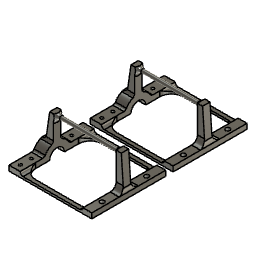
Amemometer_case v2 (Autodesk Fusion 360 design; units mm, degrees)
Autodesk Fusion 360 part; units mm, degrees
sketch "Sketch1" plane through (0, 0, 0) normal (0, 0, 1) x (1, 0, 0)
  arc A0 (0, 10) -> (0, -10) centre (0, 0) ccw
  line L0 (0, -10) -> (0, -50)
  line L1 (0, -50) -> (-7, -50)
  line L2 (-7, -50) -> (-7, -17)
  line L3 (0, 10) -> (0, 50)
  line L4 (0, 50) -> (-7, 50)
  line L5 (-7, 50) -> (-7, 17)
  line L6 (-52, -5) -> (-17.6918, -5)
  line L7 (-52, -5) -> (-52, 5)
  line L8 (-52, 5) -> (-17.6918, 5)
  arc A1 (-17.6918, -5) -> (-7, -17) centre (0, 0) ccw
  arc A2 (-7, 17) -> (-17.6918, 5) centre (0, 0) ccw
  dimension "d2" = 40
  dimension "d3" = 40
  dimension "d5" = 7
  dimension "d8" = 7
  dimension "d13" = 33
  dimension "d14" = 33
  dimension "d41" = 10
  dimension "d42" = 10
  dimension "d43" = 7
  dimension "d44" = 7
  dimension "d45" = 52
  dimension "d47" = 5
  constraint coincident A0.centre A1.centre
  constraint vertical L0
  constraint perpendicular L0 L1
  constraint perpendicular L1 L2
  constraint vertical L3
  constraint perpendicular L3 L4
  constraint perpendicular L4 L5
  constraint perpendicular L6 L7
  constraint perpendicular L2 L8
  measures "d2" distance of A0.start L3.end
  measures "d3" distance of A0.end L0.end
  measures "d5" distance of L3.end L4.end
  measures "d8" distance of L0.end L1.end
  measures "d13" distance of L4.end L5.end
  measures "d14" distance of L1.end L2.end
  measures "d41" distance of L6.start L7.end
  measures "d42" radius of A0
  measures "d43" horizontal distance of L2.end A0.centre
  measures "d44" horizontal distance of L5.end A0.centre
  measures "d45" distance of A0.centre L7
  measures "d47" vertical distance of A0.centre L6.start
extrude "Extrude1" add sketch "Sketch1" along normal blind 15 makes body 1
sketch "Sketch2" plane through (0, -5, 0) normal (0, -1, 0) x (1, 0, 0)
  line L0 (-18.9934, 15) -> (-46, 15)
  line L1 (-52, 0) -> (-17.6918, 0)
  line L2 (-17.6918, 0) -> (-17.6918, 15)
  line L3 (-17.6918, 15) -> (-52, 15)
  line L4 (-52, 15) -> (-52, 0)
  line L5 (-17.6918, 0) -> (-52, 0)
  line L6 (-52, 10) -> (-17.6918, 5)
  dimension "d52" = 10
  dimension "d53" = 5
  constraint coincident L1.end L2.start
  constraint coincident L1.start L4.end
  constraint coincident L4 L6.start
  constraint coincident L2 L6.end
  measures "d52" distance of L1.start L6.start
  measures "d53" distance of L1.end L6.end
extrude "Extrude2" cut sketch "Sketch2" against normal blind 10 contours L1 L2 L4 L5 L6 bodies 1
fillet "Fillet1" radius 4 4 edges at (-17.6918, -5, 10) (-7, -17, 7.5) (-17.6918, 5, 10) (-7, 17, 7.5) on bodies 1
fillet "Fillet2" radius 6 1 edges at (-17.6918, 0, 5) on bodies 1
sketch "Sketch3" plane through (0, 0, 15) normal (0, 0, 1) x (-1, 0, 0)
  line L0 (0, -10) -> (0, -50)
  line L1 (0, -50) -> (7, -50)
  line L2 (7, -50) -> (7, -19.4956)
  line L3 (7, 19.4956) -> (7, 50)
  line L4 (7, 50) -> (0, 50)
  line L5 (0, 50) -> (0, 10)
  arc A0 (0, -10) -> (0, 10) centre (0, 0) ccw
  circle A1 centre (48, 0) radius 2.5
  line L6 (0, 50) -> (3, 50)
  line L7 (3, 50) -> (3, 45)
  line L8 (3, 45) -> (0, 45)
  line L9 (0, 45) -> (0, 50)
  line L10 (0, -50) -> (3, -50)
  line L11 (3, -50) -> (3, -45)
  line L12 (3, -45) -> (0, -45)
  line L13 (0, -45) -> (0, -50)
  arc A2 (9.0344, -16.0119) -> (16.8334, -7.3918) centre (0, 0) ccw
  line L14 (20.4958, -5) -> (52, -5)
  line L15 (52, -5) -> (52, 5)
  line L16 (52, 5) -> (20.4958, 5)
  arc A3 (16.8334, 7.3918) -> (9.0344, 16.0119) centre (0, 0) ccw
  arc A4 (9.0344, -16.0119) -> (7, -19.4956) centre (11, -19.4956) ccw
  arc A5 (20.4958, -5) -> (16.8334, -7.3918) centre (20.4958, -9) ccw
  arc A6 (16.8334, 7.3918) -> (20.4958, 5) centre (20.4958, 9) ccw
  arc A7 (7, 19.4956) -> (9.0344, 16.0119) centre (11, 19.4956) ccw
  dimension "d35" = 5
  dimension "d36" = 3
  dimension "d37" = 5
  dimension "d38" = 5
  dimension "d39" = 3
  dimension "d50" = 4
  dimension "d51" = 5
  constraint horizontal L6
  constraint vertical L7
  constraint horizontal L8
  constraint vertical L9
  constraint coincident L4.end L5.start
  constraint horizontal L10
  constraint vertical L11
  constraint horizontal L12
  constraint vertical L13
  constraint coincident L0.end L1.start
  measures "d35" distance of L6.end L7.end
  measures "d36" distance of L7.end L8.end
  measures "d37" diameter of A1
  measures "d38" distance of L10.end L11.end
  measures "d39" distance of L11.end L12.end
  measures "d50" distance of A1.centre L15
  measures "d51" vertical distance of A1.centre L14.end
extrude "Extrude3" add sketch "Sketch3" along normal blind 85 contours L0 L1 L10 L11 L12 L13 | L4 L5 L6 L7 L8 L9 | A1 bodies 1
sketch "Sketch4" plane through (0, 0, 100) normal (0, 0, 1) x (-1, 0, 0)
  circle A0 centre (48, 0) radius 2.5
  line L0 (0, 50) -> (0, -50)
  line L1 (0, -50) -> (7, -50)
  line L2 (7, -50) -> (7, -5)
  line L3 (7, -5) -> (52, -5)
  line L4 (52, -5) -> (52, 5)
  line L5 (52, 5) -> (7, 5)
  line L6 (7, 5) -> (7, 50)
  line L7 (7, 50) -> (0, 50)
  dimension "d103" = 10
  dimension "d104" = 45
  dimension "d105" = 45
  dimension "d106" = 100
  dimension "d107" = 7
  dimension "d108" = 7
  dimension "d109" = 50
  dimension "d110" = 7
  constraint vertical L0
  constraint perpendicular L0 L1
  constraint perpendicular L1 L2
  constraint perpendicular L0 L3
  constraint perpendicular L3 L4
  constraint perpendicular L4 L5
  constraint perpendicular L5 L6
  constraint perpendicular L6 L7
  measures "d103" distance of L3.end L4.end
  measures "d104" distance of L4.end L5.end
  measures "d105" distance of L5.end L6.end
  measures "d106" distance of L0.start L0.end
  measures "d107" distance of L0.start L6.end
  measures "d108" distance of L0.end L1.end
  measures "d109" distance of origin L0.end
  measures "d110" horizontal distance of origin L2.end
extrude "Extrude4" add sketch "Sketch4" along normal blind 12 contours A0 | L0 L1 L2 L3 L4 L5 L6 L7 bodies 1
sketch "Sketch5" plane through (0, 5, 0) normal (0, 1, 0) x (-1, 0, 0)
  line L0 (7, 100) -> (52, 100)
  line L1 (52, 100) -> (52, 112)
  line L2 (52, 112) -> (7, 112)
  line L3 (7, 112) -> (7, 100)
  line L4 (7, 112) -> (52, 112)
  line L5 (52, 107) -> (7, 110)
  dimension "d62" = 5
  dimension "d63" = 2
  constraint coincident L2.end L3.start
  constraint coincident L1.end L2.start
  constraint coincident L1 L5.start
  constraint coincident L3 L5.end
  measures "d62" distance of L1.end L5.start
  measures "d63" distance of L2.end L5.end
extrude "Extrude5" cut sketch "Sketch5" against normal blind 10 contours L1 L2 L3 L4 L5 bodies 1
fillet "Fillet3" radius 8 2 edges at (-7, 5, 105) (-7, -5, 105) on bodies 1
fillet "Fillet4" radius 8 2 edges at (-7, 9, 110) (-7, -4, 110) on bodies 1
fillet "Fillet5" radius 4 4 edges at (-3, 47.5, 15) (-3, -47.5, 15) (-3, 47.5, 100) (-3, -47.5, 100) on bodies 1
fillet "Fillet6" radius 16 2 edges at (-3.5, -45, 15) (-3.5, 45, 15) on bodies 1
fillet "Fillet7" radius 8 2 edges at (-3.5, 45, 100) (-3.5, -45, 100) on bodies 1
fillet "Fillet8" radius 6 1 edges at (-45.6692, -0.904, 15) on bodies 1
fillet "Fillet9" radius 3 1 edges at (-45.6692, 0.904, 100) on bodies 1
sketch "Sketch6" plane through (0, 0, 0) normal (1, 0, 0) x (0, 1, 0)
  circle A0 centre (42, 7.5) radius 2
  circle A1 centre (-27, 7.5) radius 2
  circle A2 centre (30, 106) radius 3
  circle A3 centre (-30, 106) radius 3
  circle A4 centre (27, 7.5) radius 2
  circle A5 centre (-42, 7.5) radius 2
  point P0 (50, 0)
  point P1 (-50, 0)
  point P2 (50, 112)
  point P3 (50, 100)
  point P4 (-50, 112)
  dimension "d78" = 4
  dimension "d79" = 4
  dimension "d80" = 6
  dimension "d81" = 6
  dimension "d82" = 4
  dimension "d83" = 4
  dimension "d88" = 7.5
  dimension "d89" = 23
  dimension "d90" = 7.5
  dimension "d91" = 8
  dimension "d92" = 7.5
  dimension "d93" = 7.5
  dimension "d94" = 23
  dimension "d95" = 8
  measures "d78" diameter of A0
  measures "d79" diameter of A1
  measures "d80" diameter of A2
  measures "d81" diameter of A3
  measures "d82" diameter of A4
  measures "d83" diameter of A5
  measures "d88" vertical distance of A0.centre P0
  measures "d89" horizontal distance of A4.centre P0
  measures "d90" vertical distance of A4.centre P0
  measures "d91" horizontal distance of A0.centre P0
  measures "d92" vertical distance of A5.centre P1
  measures "d93" vertical distance of A1.centre P1
  measures "d94" horizontal distance of A1.centre P1
  measures "d95" horizontal distance of A5.centre P1
extrude "Extrude6" cut sketch "Sketch6" against normal blind 10 bodies 1
move_body "Move1" bodies 1 to x (1, 0, 0) y (0, 1, 0) z (0, 0, 1) at (-5, 0, 0)
move_body "Move2" bodies 1 to x (0, 0, -1) y (0, 1, 0) z (1, 0, 0) at (-5, 0, -5)
move_body "Move3" bodies 1 to x (1, 0, 0) y (0, 1, 0) z (0, 0, 1) at (10, 55, 0)
mirror "Mirror2" about plane through (0, 0, 0) normal (0, 1, 0) of bodies 1 makes body 2
